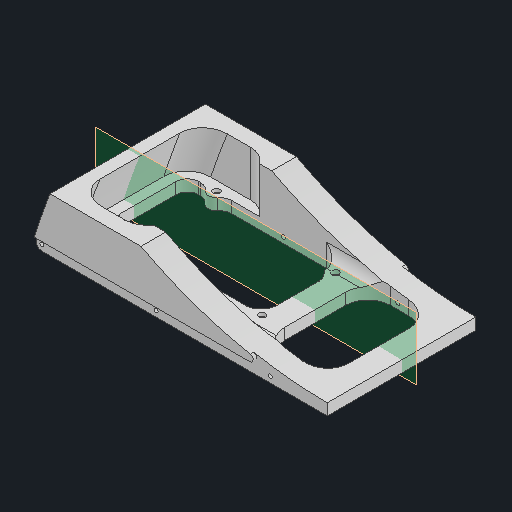
# Autodesk Inventor part: bottom_front_01
Saved by Autodesk Inventor 2022 (Build 260153000, 153)
## iProperties
Created: 2025-01-09
Part Number: bottom_front_01
Material: 一般
Document SubType Name: Modeling
Designer: nyxeon
Density: 1 g/cm^3
Appearance: 既定
Author: nyxeon
Autodesk Inventor part; units mm, degrees
ref_plane "YZ Plane" through (0, 0, 0) normal (1, 0, 0) x (0, 1, 0)
ref_plane "XZ Plane" through (0, 0, 0) normal (0, 1, 0) x (-1, 0, 0)
ref_plane "XY Plane" through (0, 0, 0) normal (0, 0, 1) x (1, 0, 0)
sketch "スケッチ2" plane through (0, 0, 0) normal (0, 0, 1) x (1, 0, 0)
  circle A0 centre (-250, 200) radius 2.1 construction
  circle A1 centre (-150, 200) radius 2.1 construction
  circle A2 centre (-50, 200) radius 2.1 construction
  circle A3 centre (50, 200) radius 2.1 construction
  line L0 (-50, 200) -> (50, 200) construction
  line L1 (0, 200) -> (0, 245) construction
  line L2 (-359.920454, 245) -> (374.522722, 245) construction
  line L3 (250, 205) -> (-250, 205) construction
  circle A4 centre (-250, 200) radius 5 construction
  circle A5 centre (-150, 200) radius 5 construction
  circle A6 centre (-50, 200) radius 5 construction
  line L4 (-255, 200) -> (-255, -200) construction
  line L5 (-255, 200) -> (-255, 245) construction
  line L6 (-250, 195) -> (-0.1, 195)
  line L7 (-0.1, 195) -> (-0.1, 205)
  line L8 (-145, 200) -> (-145, 245) construction
  circle A7 centre (-50, 200) radius 1.75
  circle A8 centre (-150, 200) radius 1.75
  circle A9 centre (-250, 200) radius 1.75
  arc A10 (-239.805165, 245) -> (-285, 0) centre (401.666667, 0) ccw
  line L9 (-150, 200) -> (-250, 200) construction
  line L10 (-200, 200) -> (-200, 245) construction
  arc A11 (-160.194835, 245) -> (-0.1, 205) centre (0, 545.779689) ccw
  line L11 (-160.194835, 245) -> (-239.805165, 245)
  arc A12 (-254.779951, 201.466993) -> (-250, 195) centre (-250, 200) ccw
  point P0 (0, 0)
  dimension "d0" = 0.1
  dimension "d1" = 3.5
  dimension "d2" = 30
  dimension "d3" = 39.80517
  dimension "d4" = 39.80517
  constraints: 20 end point, 10 point on circle, 8 centre point, 7 coincident, 6 point on line, 5 horizontal alignment, 4 perpendicular, 4 tangent, 3 horizontal, 2 equal radius, 2 midpoint, 2 parallel, 2 vertical, 1 collinear, 1 vertical alignment, 4 other
  measures "d0" distance between parallel lines of L1 L7
  measures "d1" diameter of A7
  measures "d2" distance from line of L4 A10.end
  measures "d3" distance of L11.end L10.end
  measures "d4" distance from line of A11.start L10
extrude "押し出し1" add sketch "スケッチ2" along normal blind 130 contours A12 A10 L11 A11 L7 L6 | A7 | A8 | A9
shell "シェル1" thickness 10 removed faces 2 at (-186.731612, 245, 43.333333) at (-131.519967, 231.402042, 86.666667)
sketch "スケッチ3" plane through (-250, 195, 0) normal (0, -1, 0) x (1, 0, 0)
  circle A0 centre (17, 92.166373) radius 1.25 construction
  circle A1 centre (41, 18.166373) radius 1.25 construction
  circle A2 centre (155, 92.166373) radius 1.25 construction
  circle A3 centre (155, 28.166373) radius 1.25 construction
  circle A4 centre (155, 92.166373) radius 1.8
  circle A5 centre (155, 28.166373) radius 1.8
  circle A6 centre (17, 92.166373) radius 1.8
  circle A7 centre (41, 18.166373) radius 1.8
  arc A8 (158.8, 12.566373) -> (160, 13.766373) centre (158.8, 13.766373) ccw construction
  arc A9 (11.2, 97.966373) -> (10, 96.766373) centre (11.2, 96.766373) ccw construction
  line L0 (160, 97.966373) -> (10, 97.966373) construction
  line L1 (10, 97.966373) -> (10, 12.566373) construction
  line L2 (10, 12.566373) -> (160, 12.566373) construction
  line L3 (160, 12.566373) -> (160, 97.966373) construction
  line L4 (154, 91.966373) -> (16, 91.966373) construction
  line L5 (16, 91.966373) -> (16, 18.566373) construction
  line L6 (16, 18.566373) -> (154, 18.566373) construction
  line L7 (154, 18.566373) -> (154, 91.966373) construction
  circle A10 centre (155, 92.166373) radius 7 construction
  circle A11 centre (155, 28.166373) radius 7 construction
  circle A12 centre (17, 92.166373) radius 7 construction
  circle A13 centre (41, 18.166373) radius 7 construction
  arc A14 (148.002858, 91.966373) -> (154, 85.23817) centre (155, 92.166373) ccw
  arc A15 (154, 35.094576) -> (154, 21.23817) centre (155, 28.166373) ccw
  arc A16 (47.988562, 18.566373) -> (34.011438, 18.566373) centre (41, 18.166373) ccw
  arc A17 (16, 85.23817) -> (23.997142, 91.966373) centre (17, 92.166373) ccw
  line L8 (16, 85.23817) -> (16, 18.566373)
  line L9 (34.011438, 18.566373) -> (16, 18.566373)
  line L10 (23.997142, 91.966373) -> (148.002858, 91.966373)
  line L11 (154, 85.23817) -> (154, 35.094576)
  line L12 (154, 21.23817) -> (154, 18.566373)
  line L13 (154, 18.566373) -> (47.988562, 18.566373)
  point P0 (250, 0)
  dimension "d9" = 3.6
  dimension "d10" = 6
  dimension "d11" = 14
  constraints: 28 end point, 16 point on circle, 13 point on line, 12 centre point, 12 coincident, 6 equal radius, 4 parallel, 3 collinear, 3 perpendicular, 2 horizontal, 3 other
  measures "d9" diameter of A4
  measures "d10" distance between parallel lines of L3 L7
  measures "d11" diameter of A10
extrude "押し出し2" cut sketch "スケッチ3" against normal through all
sketch "スケッチ4" plane through (0, 0, 0) normal (0, 0, -1) x (-1, 0, 0)
  circle A0 centre (250, 200) radius 2.1 construction
  circle A1 centre (150, 200) radius 2.1 construction
  circle A2 centre (50, 200) radius 2.1 construction
  circle A3 centre (250, 200) radius 1.75
  circle A4 centre (150, 200) radius 1.75
  circle A5 centre (50, 200) radius 1.75
  point P0 (0, 0)
  dimension "d14" = 3.5
  constraints: 3 centre point, 3 coincident, 2 equal radius
  measures "d14" diameter of A3
extrude "押し出し3" cut sketch "スケッチ4" against normal through all
sketch "スケッチ5" plane through (-243.199814, 205, 10) normal (0, 0, 1) x (1, 0, 0)
  arc A0 (14.110761, 40) -> (0, 0) centre (644.866481, -205) ccw
  line L0 (83.004979, 40) -> (3.394649, 40)
  arc A1 (3.394649, 40) -> (-11.580137, -3.533007) centre (644.866481, -205) ccw
  line L1 (0, 0) -> (233.099814, 0)
  line L2 (0, 0) -> (-10.485418, 0)
  point P0 (243.199814, -205)
  constraints: 2 end point, 1 horizontal, 1 point on circle
extrude "押し出し4" add sketch "スケッチ5" along normal up to surface (110 mm away)
sketch "スケッチ6" plane through (-243.199814, 205, 120) normal (0, 1, 0) x (1, 0, 0)
  circle A0 centre (10.199814, 27.833627) radius 1.8 construction
  circle A1 centre (34.199814, 101.833627) radius 1.8 construction
  circle A2 centre (148.199814, 91.833627) radius 1.8 construction
  circle A3 centre (148.199814, 27.833627) radius 1.8 construction
  circle A4 centre (10.199814, 27.833627) radius 3
  circle A5 centre (148.199814, 27.833627) radius 3
  circle A6 centre (148.199814, 91.833627) radius 3
  circle A7 centre (34.199814, 101.833627) radius 3
  point P0 (243.199814, 120)
  dimension "d19" = 6
  constraints: 4 centre point, 4 coincident, 3 equal radius
  measures "d19" diameter of A4
extrude "押し出し5" cut sketch "スケッチ6" against normal blind 3
fillet "フィレット1" radius 10 10 edges at (-226.0029, 200, 91.9664) (-234, 200, 85.2382) (-234, 200, 18.5664) (-215.9886, 200, 18.5664) (-202.0114, 200, 18.5664) (-96, 200, 18.5664) (-96, 200, 21.2382) (-96, 200, 35.0946) (-96, 200, 85.2382) (-101.9971, 200, 91.9664)
sketch "スケッチ7" plane through (0, 0, 0) normal (0, 0, -1) x (-1, 0, 0)
  circle A0 centre (50, 200) radius 1.75
  circle A1 centre (150, 200) radius 1.75
  circle A2 centre (250, 200) radius 1.75
  line L0 (0.1, 195) -> (0.1, 205)
  line L1 (250, 195) -> (0.1, 195)
  arc A3 (250, 195) -> (254.779951, 201.466993) centre (250, 200) ccw
  arc A4 (254.779951, 201.466993) -> (239.805165, 245) centre (-401.666667, 0) ccw
  line L2 (160.194835, 245) -> (239.805165, 245)
  arc A5 (0.1, 205) -> (160.194835, 245) centre (0, 545.779689) ccw
  line L3 (250, 205) -> (-250, 205) construction
  arc A6 (254.779951, 201.466993) -> (239.805165, 245) centre (-401.666667, 0) ccw construction
  line L4 (253.622637, 205.2) -> (11.673983, 205.2)
  arc A7 (0.1, 205) -> (160.194835, 245) centre (0, 545.779689) ccw construction
  point P0 (0, 0)
  dimension "d23" = 0.2
  constraints: 2 end point, 2 point on circle, 1 horizontal
  measures "d23" distance between parallel lines of L4 L3
extrude "押し出し6" add sketch "スケッチ7" along normal blind 3 contours A5 L2 A4 L4
sketch "スケッチ8" plane through (0, 0, 130) normal (0, 0, 1) x (1, 0, 0)
  arc A0 (-160.194835, 245) -> (-11.673983, 205.2) centre (0, 545.779689) ccw
  line L0 (-11.673983, 205.2) -> (-253.622637, 205.2)
  arc A1 (-239.805165, 245) -> (-253.622637, 205.2) centre (401.666667, 0) ccw
  line L1 (-239.805165, 245) -> (-160.194835, 245)
  point P0 (0, 0)
extrude "押し出し7" add sketch "スケッチ8" along normal blind 3
fillet "フィレット2" radius 20 2 edges at (-236.4579, 225.1106, 10) (-236.4579, 225.1106, 120)
sketch "スケッチ9" plane through (-222.18116, 205, 10) normal (0, 0, 1) x (1, 0, 0)
  arc A0 (14.597377, 40) -> (0, 0) centre (623.847827, -205) ccw
  line L0 (0, 0) -> (212.08116, 0)
  line L1 (212.08116, 0) -> (212.08116, 0.14969)
  arc A1 (61.986325, 40) -> (212.08116, 0.14969) centre (222.18116, 340.779689) ccw
  line L2 (14.597377, 40) -> (61.986325, 40)
  line L3 (14.597377, 40) -> (61.986325, 40)
  line L4 (51.270213, 40) -> (51.270213, 0)
  line L5 (0, 0) -> (212.08116, 0)
  point P0 (222.18116, -205)
  point P1 (-6.907893, 40)
  point P2 (-17.624005, 40)
  point P3 (51.270213, 40)
  dimension "d29" = 10.71611
  dimension "d30" = 10.71611
  constraints: 2 end point, 2 point on line, 1 perpendicular
  measures "d29" distance of point (-17.624, 40) point (-6.908, 40)
  measures "d30" distance of L2.end L4.start
extrude "押し出し8" add sketch "スケッチ9" along normal up to surface (8.566373 mm away) contours L2 A1 L1 L0 L4
fillet "フィレット3" radius 20 1 edges at (-170.9109, 225, 10)
ref_plane "作業平面2" through (0, 0, 65) normal (0, 0, -1) x (-1, 0, 0)
mirror "ミラー1" about plane through (0, 0, 65) normal (0, 0, -1) of "押し出し8", "フィレット3"
sketch "スケッチ10" plane through (-219.4, 205, 91.966373) normal (0, 1, 0) x (1, 0, 0)
  line L0 (209.3, -19.467254) -> (59.205165, -19.467254) construction
  line L1 (209.3, 73.4) -> (59.205165, 73.4) construction
  line L2 (219.3, 91.966373) -> (219.3, -38.033627) construction
  line L3 (199.3, -19.467254) -> (143.4, -19.467254)
  line L4 (143.4, -19.467254) -> (143.4, 73.4)
  line L5 (143.4, 73.4) -> (199.3, 73.4)
  line L6 (199.3, 73.4) -> (199.3, -19.467254)
  line L7 (123.4, 50.838519) -> (123.4, 12.761481) construction
  point P0 (219.4, 91.966373)
  dimension "d34" = 20
  dimension "d35" = 20
  constraints: 8 end point, 2 parallel, 2 point on line, 1 horizontal, 1 perpendicular
  measures "d34" distance between parallel lines of L6 L2
  measures "d35" distance between parallel lines of L7 L4
extrude "押し出し9" cut sketch "スケッチ10" along normal through all both and the other way through all
sketch "スケッチ11" plane through (-160.194835, 245, 111.433627) normal (0, 0, -1) x (-1, 0, 0)
  circle A0 centre (-110.194835, -45) radius 1.75
  line L0 (10.716112, -40) -> (-84.194835, -40)
  line L1 (10.716112, 0) -> (10.716112, -40)
  line L2 (0, 0) -> (10.716112, 0)
  arc A1 (-150.094835, -39.85031) -> (0, 0) centre (-160.194835, 300.779689) ccw
  line L3 (-150.094835, -40) -> (-150.094835, -39.85031)
  line L4 (-140.094835, -40) -> (-150.094835, -40)
  line L5 (-140.094835, -50) -> (-140.094835, -40)
  line L6 (-84.194835, -50) -> (-140.094835, -50)
  line L7 (-84.194835, -50) -> (-84.194835, -40)
  line L8 (-140.094835, -50) -> (-140.094835, -40)
  line L9 (-140.094835, -40) -> (-140.094835, -39.406725)
  point P0 (-160.194835, -245)
  constraints: 2 end point, 1 point on circle, 1 point on line
extrude "押し出し10" add sketch "スケッチ11" along normal up to surface (92.867254 mm away) contours L9 L4 L3 A1
fillet "フィレット4" radius 20 4 edges at (-20.1, 200.2966, 111.4336) (-76, 200, 111.4336) (-20.1, 200.2966, 18.5664) (-76, 200, 18.5664)
fillet "フィレット5" radius 10 4 edges at (-66, 205, 18.5664) (-93.9976, 205, 18.5664) (-66, 205, 111.4336) (-123.4555, 205, 111.4336)
fillet "フィレット6" radius 3 2 edges at (-11.674, 205.2, -1.5) (-11.674, 205.2, 131.5)
equation "\"d4\" = d3"
equation "\"d30\" = d29"
